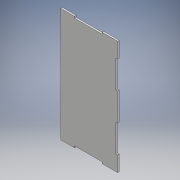
# Autodesk Inventor part: Piso
Saved by Autodesk Inventor 2018 (Build 220112000, 112)
## iProperties
Created: 2020-03-11
Part Number: Piso
Material: Genérico
Document SubType Name: Modeling
Designer: joser
Density: 1 g/cm^3
Appearance: Valor por defecto
Author: joser
Autodesk Inventor part; units mm, degrees
ref_plane "YZ Plane" through (0, 0, 0) normal (1, 0, 0) x (0, 1, 0)
ref_plane "XZ Plane" through (0, 0, 0) normal (0, 1, 0) x (-1, 0, 0)
ref_plane "XY Plane" through (0, 0, 0) normal (0, 0, 1) x (1, 0, 0)
sketch "Boceto1" plane through (0, 0, 0) normal (0, 1, 0) x (-1, 0, 0)
  line L0 (51.5, 103) -> (51.5, -103)
  line L1 (-51.5, 103) -> (51.5, -103) construction
  line L2 (51.5, 103) -> (-51.5, -103) construction
  line L3 (26.5, 103) -> (26.5, 100)
  line L4 (26.5, 100) -> (-23.5, 100)
  line L5 (-23.5, 100) -> (-23.5, 103)
  line L6 (-51.5, 103) -> (-23.5, 103)
  line L7 (26.5, 103) -> (51.5, 103)
  line L8 (26.5, -103) -> (26.5, -100)
  line L9 (26.5, -100) -> (-23.5, -100)
  line L10 (-23.5, -100) -> (-23.5, -103)
  line L11 (51.5, -103) -> (26.5, -103)
  line L12 (-23.5, -103) -> (-51.5, -103)
  line L13 (-51.5, 75) -> (-48.5, 75)
  line L14 (-48.5, 75) -> (-48.5, 25)
  line L15 (-48.5, 25) -> (-51.5, 25)
  line L16 (-51.5, 75) -> (-51.5, 103)
  line L17 (-51.5, -25) -> (-48.5, -25)
  line L18 (-48.5, -25) -> (-48.5, -75)
  line L19 (-48.5, -75) -> (-51.5, -75)
  line L20 (-51.5, -103) -> (-51.5, -75)
  line L21 (-51.5, -25) -> (-51.5, 25)
  point P0 (0, 0)
  dimension "d4" = 3
  dimension "d5" = 50
  dimension "d7" = 3
  dimension "d8" = 50
  dimension "d24" = 50
  dimension "d30" = 3
  dimension "d33" = 25
  dimension "d35" = 100
  dimension "d36" = 25
  dimension "d38" = 200
  constraints: 44 end point, 15 perpendicular, 8 parallel, 5 collinear, 3 equal length, 3 horizontal, 2 midpoint, 2 vertical
  measures "d4" distance of L3.start L3.end
  measures "d5" distance of L3.end L4.end
  measures "d7" distance of L8.start L8.end
  measures "d8" distance of L8.end L9.end
  measures "d24" distance of L13.end L14.end
  measures "d30" distance between parallel lines of L16 L14
  measures "d33" distance between parallel lines of L4 L13
  measures "d35" distance between parallel lines of L0 L18
  measures "d36" distance between parallel lines of L5 L14
  measures "d38" distance between parallel lines of L4 L9
extrude "Extrusión1" add sketch "Boceto1" along normal blind 3
